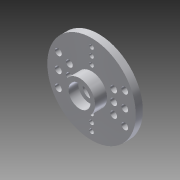
# Autodesk Inventor part: servo arm DS939HV round
Saved by Autodesk Inventor 2013 (Build 170138000, 138)
## iProperties
Created: 2014-10-08
Part Number: servo arm DS939HV round
Material: Generic
Document SubType Name: Modeling
Designer: Masta
Density: 1 g/cm^3
Author: Masta
Autodesk Inventor part; units mm, degrees
ref_plane "YZ Plane" through (0, 0, 0) normal (1, 0, 0) x (0, 1, 0)
ref_plane "XZ Plane" through (0, 0, 0) normal (0, 1, 0) x (-1, 0, 0)
ref_plane "XY Plane" through (0, 0, 0) normal (0, 0, 1) x (1, 0, 0)
sketch "Sketch1" plane through (0, 0, 0) normal (0, 1, 0) x (-1, 0, 0)
  circle A0 centre (0, 0) radius 3.5
  circle A1 centre (0, 0) radius 10
  line L0 (0, 0) -> (-7.5, 0) construction
  line L1 (0, 0) -> (0, 3.5) construction
  line L2 (0, 3.5) -> (0, 10) construction
  point P0 (-5, 0)
  point P1 (-7.5, 3.5)
  point P2 (-5, 2.5)
  point P3 (0, 4.75)
  dimension "d0" = 7
  dimension "d2" = 20
  dimension "d3" = 7.5
  dimension "d47" = 5
  dimension "d50" = 3.5
  dimension "d57" = 2.5
  dimension "d62" = 4.75
  constraints: 6 end point, 2 coincident, 2 point on line, 2 vertical, 2 vertical alignment, 1 collinear, 1 horizontal, 1 perpendicular, 6 other
  measures "d3" distance of L0.start L0.end
  measures "d47" distance of point (0, 0) point (-5, 0)
  measures "d50" distance of point (-7.5, 0) point (-7.5, 3.5)
  measures "d57" distance of point (-5, 0) point (-5, 2.5)
  measures "d62" distance of point (0, 4.75) point (0, 0)
extrude "Extrusion1" add sketch "Sketch1" along normal blind 1.6 contours A0 | A1
extrude "Extrusion2" add sketch "Sketch1" against normal blind 2.7 and the other way blind 2 contours A0
hole "Hole2" at (0, -2.7, 0) direction (0, 1, 0) diameter 3 end through all
hole "Hole3" at (0, -2.7, 0) direction (0, 1, 0) diameter 5 depth 2.2
hole "Hole5" at (0, 2, 0) direction (0, -1, 0) diameter 5 depth 0.8
hole "Hole6" at (7.5, 0, 0) at (5, 0, 0) at (7.5, 0, 3.5) at (5, 0, 2.5) direction (0, 1, 0) diameter 1.5 end through all
mirror "Mirror1" about plane through (0, 0, 0) normal (1, 0, 0) of "Hole6"
hole "Hole7" at (0, 0, 4.75) direction (0, 1, 0) diameter 1 end through all
pattern_linear "Rectangular Pattern1" count 3 spacing 1.75 along (0, 0, 1) of "Hole7"
mirror "Mirror2" about plane through (0, 0, 0) normal (0, 0, 1) of "Hole6", "Mirror1", "Hole7", "Rectangular Pattern1"
body "Solid1"
